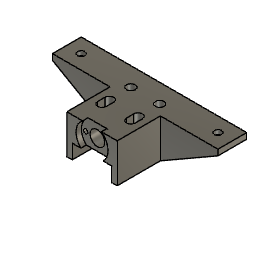
Z Carriage Bracket (Autodesk Fusion 360 design; units mm, degrees)
Autodesk Fusion 360 part; units mm, degrees
sketch "Sketch1" plane through (0, 0, 0) normal (0, 0, 1) x (1, 0, 0)
  line L0 (17.5, 25) -> (-17.5, 25)
  line L1 (-17.5, 25) -> (-17.5, -25)
  line L2 (-17.5, -25) -> (17.5, -25)
  line L3 (17.5, -25) -> (17.5, 25)
  line L4 (17.5, 25) -> (-17.5, -25) construction
  line L5 (-17.5, 25) -> (17.5, -25) construction
  line L6 (-13.7, 25) -> (13.7, 25)
  line L7 (13.7, 25) -> (13.7, -25)
  line L8 (13.7, -25) -> (-13.7, -25)
  line L9 (-13.7, -25) -> (-13.7, 25)
  line L10 (-57.5, 25) -> (57.5, 25)
  line L11 (57.5, 25) -> (57.5, 5)
  line L12 (57.5, 5) -> (-57.5, 5)
  line L13 (-57.5, 5) -> (-57.5, 25)
  line L14 (17.5, -8) -> (-17.5, -8) construction
  line L15 (17.5, 12) -> (-17.5, 12) construction
  line L16 (-10, -25) -> (-10, 25) construction
  line L17 (10, -25) -> (10, 26.6131) construction
  circle A0 centre (10, -8) radius 1.5
  circle A1 centre (10, 12) radius 1.5
  circle A2 centre (-10, 12) radius 1.5
  circle A3 centre (-10, -8) radius 1.5
  circle A4 centre (10, 12) radius 3
  circle A5 centre (-10, 12) radius 3
  circle A6 centre (-10, -8) radius 3
  circle A7 centre (10, -8) radius 3
  circle A8 centre (47.5, 15) radius 2.5
  circle A9 centre (47.5, 15) radius 4.5
  circle A10 centre (-47.5, 15) radius 2.5
  circle A11 centre (-47.5, 15) radius 4.5
  line L18 (-17.5, 21) -> (-57.5, 21)
  line L19 (-57.5, 21) -> (-57.5, 9)
  line L20 (-57.5, 9) -> (-17.5, 9)
  line L21 (-17.5, 9) -> (-17.5, 21)
  line L22 (57.5, 9) -> (17.5, 9)
  line L23 (17.5, 9) -> (17.5, 21)
  line L24 (17.5, 21) -> (57.5, 21)
  line L25 (57.5, 21) -> (57.5, 9)
  circle A12 centre (10, -3) radius 1.5
  circle A13 centre (10, -3) radius 3
  circle A14 centre (-10, -3) radius 3
  circle A15 centre (-10, -3) radius 1.5
  line L26 (-13, -8) -> (-13, -3)
  line L27 (-7, -8) -> (-7, -3)
  line L28 (7, -8) -> (7, -3)
  line L29 (13, -8) -> (13, -3)
  point P0 (-47.5, 15)
  point P1 (47.5, 15)
  dimension "d1" = 35
  dimension "d2" = 50
  dimension "d5" = 27.4
  dimension "d6" = 50
  dimension "d7" = 3.8
  dimension "d10" = 115
  dimension "d11" = 20
  dimension "d12" = 40
  dimension "d16" = 7.5
  dimension "d17" = 7.5
  dimension "d19" = 13
  dimension "d20" = 3
  dimension "d21" = 3
  dimension "d22" = 3
  dimension "d23" = 3
  dimension "d30" = 6
  dimension "d31" = 6
  dimension "d32" = 6
  dimension "d33" = 6
  dimension "d40" = 5
  dimension "d41" = 9
  dimension "d42" = 5
  dimension "d43" = 9
  dimension "d52" = 40
  dimension "d53" = 12
  dimension "d54" = 12
  dimension "d71" = 20
  dimension "d81" = 10
  dimension "d82" = 10
  dimension "d83" = 10
  dimension "d84" = 10
  dimension "d94" = 3
  dimension "d95" = 3
  dimension "d96" = 6
  dimension "d97" = 6
  dimension "d98" = 5
  constraint perpendicular L0 L1
  constraint parallel L0 L2
  constraint parallel L1 L3
  constraint horizontal L0
  constraint coincident L4 origin
  constraint coincident L5 origin
  constraint horizontal L6
  constraint vertical L7
  constraint horizontal L8
  constraint vertical L9
  constraint coincident L0 L6.start
  constraint horizontal L10
  constraint vertical L11
  constraint horizontal L12
  constraint vertical L13
  constraint coincident L0 L10.start
  constraint coincident L3 L14.start
  constraint coincident L1 L14.end
  constraint perpendicular L1 L14
  constraint coincident L3 L15.start
  constraint coincident L1 L15.end
  constraint perpendicular L1 L15
  constraint coincident L2 L16.start
  constraint coincident L0 L16.end
  constraint coincident L8 L17.start
  constraint perpendicular L10 L17
  constraint coincident L14 A0.centre
  constraint coincident L17 A0.centre
  constraint coincident L17 A1.centre
  constraint coincident L15 A1.centre
  constraint coincident L15 A2.centre
  constraint coincident L16 A2.centre
  constraint coincident L14 A3.centre
  constraint coincident L16 A3.centre
  constraint concentric A1 A4
  constraint concentric A2 A5
  constraint concentric A3 A6
  constraint concentric A0 A7
  constraint concentric A8 A9
  constraint concentric A10 A11
  constraint perpendicular L18 L19
  constraint parallel L18 L20
  constraint parallel L19 L21
  constraint horizontal L18
  constraint coincident P0 A10.centre
  constraint perpendicular L22 L23
  constraint parallel L22 L24
  constraint parallel L23 L25
  constraint horizontal L22
  constraint coincident P1 A8.centre
  constraint coincident L11 L22.start
  constraint concentric A14 A15
  constraint concentric A12 A13
  constraint coincident A6 L26.start
  constraint coincident L14 L26.start
  constraint coincident A14 L26.end
  constraint tangent A14 L26
  constraint perpendicular L14 L26
  constraint coincident A6 L27.start
  constraint coincident L14 L27.start
  constraint coincident A14 L27.end
  constraint tangent A14 L27
  constraint perpendicular L14 L27
  constraint coincident A7 L28.start
  constraint coincident L14 L28.start
  constraint coincident A13 L28.end
  constraint tangent A13 L28
  constraint perpendicular L14 L28
  constraint coincident A7 L29.start
  constraint coincident L14 L29.start
  constraint coincident A13 L29.end
  constraint tangent A13 L29
  constraint perpendicular L14 L29
  constraint horizontal A14.centre A12.centre
  measures "d1" distance of L1.end L2.end
  measures "d2" distance of L0.end L1.end
  measures "d5" distance of L6.start L6.end
  measures "d6" distance of L6.start L8.end
  measures "d7" distance of L1 L9
  measures "d10" distance of L10.start L10.end
  measures "d11" distance of L10.start L12.end
  measures "d12" distance of L3 L11
  measures "d16" distance of L3 L17
  measures "d17" distance of L1 L16
  measures "d19" distance of L10 L15
  measures "d20" diameter of A0
  measures "d21" diameter of A1
  measures "d22" diameter of A2
  measures "d23" diameter of A3
  measures "d30" diameter of A4
  measures "d31" diameter of A5
  measures "d32" diameter of A6
  measures "d33" diameter of A7
  measures "d40" diameter of A8
  measures "d41" diameter of A9
  measures "d42" diameter of A10
  measures "d43" diameter of A11
  measures "d52" distance of L19.end L20.end
  measures "d53" distance of L18.end L19.end
  measures "d54" distance of L22.end L23.end
  measures "d71" distance of L14 L15
  measures "d81" distance of L13 P0
  measures "d82" distance of L11 P1
  measures "d83" distance of L10 P1
  measures "d84" distance of L10 P0
  measures "d94" diameter of A12
  measures "d95" diameter of A15
  measures "d96" diameter of A14
  measures "d97" diameter of A13
  measures "d98" distance of A0.centre A12.centre
extrude "Extrude1" add sketch "Sketch1" along normal blind 27 contours L0 L3 L7 L10 L12 L23 | L0 L6 L7 L9 L10 L12 | L0 L1 L9 L10 L12 L21 | L2 L3 L7 L12 | L2 L7 L8 L9 L12 | L1 L2 L9 L12 | A0 | A1 | A2 | A3 | A4 | A5 | A6 A14 | A6 A14 L26 | A6 A14 L27 | A6 A14 | A6 A14 | A7 A13 | A7 A13 L28 | A7 A13 L29 | A7 A13 | A7 A13 | A12 | A15
extrude "Extrude2" cut sketch "Sketch1" along normal blind 10 contours L0 L6 L7 L9 L10 L12 | L2 L7 L8 L9 L12 | A0 | A1 | A2 | A3 | A4 | A5 | A6 A14 | A6 A14 L26 | A6 A14 L27 | A6 A14 | A6 A14 | A7 A13 | A7 A13 L28 | A7 A13 L29 | A7 A13 | A7 A13 | A12 | A15
extrude "Extrude3" add sketch "Sketch1" along normal blind 4 from surface at 23 contours L0 L3 L7 L10 L12 L23 | L3 L10 L11 L24 | L0 L6 L7 L9 L10 L12 | L3 L11 L22 L23 L24 L25 | L0 L1 L9 L10 L12 L21 | L3 L11 L12 L22 | L1 L10 L13 L18 | L1 L13 L18 L19 L20 L21 | L1 L12 L13 L20 | A1 | A2 | A4 | A5 | A8 | A9 | A10 | A11
extrude "Extrude6" cut sketch "Sketch1" along normal up to surface (13 mm away) from surface at 14 contours A0 | A3 | A6 A14 | A6 A14 L26 | A6 A14 L27 | A6 A14 | A6 A14 | A7 A13 | A7 A13 L28 | A7 A13 L29 | A7 A13 | A7 A13 | A12 | A15
extrude "Extrude7" cut sketch "Sketch1" along normal up to surface (13 mm away) from surface at 14 contours A1 | A2 | A4 | A5
extrude "Extrude4" cut sketch "Sketch1" along normal blind 3.8 from surface at 10 contours A0 | A3 | A12 | A15
extrude "Extrude5" cut sketch "Sketch1" along normal blind 3.8 from surface at 10 contours A1 | A2
extrude "Extrude8" cut sketch "Sketch1" along normal up to surface (4 mm away) from surface at 23 contours A8 | A10
extrude "Extrude9" cut sketch "Sketch1" along normal blind 1 from surface at 23 contours A8 | A9 | A10 | A11
extrude "Extrude10" add sketch "Sketch1" along normal up to surface (23 mm away) contours L3 L10 L11 L24 | L3 L11 L22 L23 L24 L25 | L3 L11 L12 L22 | L1 L10 L13 L18 | L1 L13 L18 L19 L20 L21 | L1 L12 L13 L20
sketch "Sketch2" plane through (0, -25, 0) normal (0, -1, 0) x (1, 0, 0)
  line L0 (-17.5, 0) -> (-17.5, 23)
  line L1 (17.5, 23) -> (17.5, 0)
  line L2 (-13.7, 0) -> (-13.7, 10)
  line L3 (-13.7, 10) -> (13.7, 10)
  line L4 (13.7, 10) -> (13.7, 0)
  line L5 (13.7, 0) -> (17.5, 0)
  line L6 (17.5, 0) -> (17.5, 27)
  line L7 (17.5, 27) -> (-17.5, 27)
  line L8 (-17.5, 27) -> (-17.5, 0)
  line L9 (-17.5, 0) -> (-13.7, 0)
  line L10 (17.5, 18) -> (-17.5, 18) construction
  line L11 (0, 23) -> (0, 10) construction
  circle A0 centre (0, 18) radius 5.125
  circle A1 centre (0, 18) radius 11.125
  line L12 (11.125, 18) -> (5.125, 18)
  line L13 (11.125, 18) -> (5.125, 18) construction
  line L14 (-5.125, 18) -> (-11.125, 18) construction
  circle A2 centre (-8.125, 18) radius 1.5
  circle A3 centre (8.125, 18) radius 1.5
  line L15 (-17.5, 27) -> (-57.5, 27)
  line L16 (-57.5, 27) -> (-57.5, 0)
  line L17 (-57.5, 0) -> (-17.5, 0)
  line L18 (-17.5, 0) -> (-17.5, 27)
  line L19 (17.5, 27) -> (57.5, 27)
  line L20 (57.5, 27) -> (57.5, 0)
  line L21 (57.5, 0) -> (17.5, 0)
  line L22 (17.5, 0) -> (17.5, 27)
  line L23 (-57.5, 27) -> (-17.5, 0) construction
  line L24 (-17.5, 27) -> (-57.5, 0) construction
  line L25 (17.5, 0) -> (57.5, 27) construction
  line L26 (17.5, 27) -> (57.5, 0) construction
  line L27 (-17.5, 23) -> (-57.5, 23)
  line L28 (-57.5, 23) -> (-57.5, 4)
  line L29 (-57.5, 4) -> (-17.5, 4)
  line L30 (-17.5, 4) -> (-17.5, 23)
  line L31 (-17.5, 23) -> (-57.5, 4) construction
  line L32 (-57.5, 23) -> (-17.5, 4) construction
  line L33 (57.5, 23) -> (17.5, 23)
  line L34 (17.5, 23) -> (17.5, 4)
  line L35 (17.5, 4) -> (57.5, 4)
  line L36 (57.5, 4) -> (57.5, 23)
  line L37 (57.5, 23) -> (17.5, 4) construction
  line L38 (17.5, 23) -> (57.5, 4) construction
  line L39 (-17.5, 0) -> (-57.5, 23)
  line L40 (17.5, 0) -> (57.5, 23)
  point P0 (-37.5, 13.5)
  point P1 (37.5, 13.5)
  dimension "d64" = 8
  dimension "d65" = 10.25
  dimension "d66" = 22.25
  dimension "d74" = 3
  dimension "d75" = 3
  dimension "d85" = 40
  dimension "d86" = 27
  dimension "d87" = 40
  dimension "d88" = 27
  dimension "d89" = 19
  dimension "d90" = 40
  dimension "d91" = 19
  constraint coincident L1 L10.start
  constraint coincident L8 L10.end
  constraint perpendicular L8 L10
  constraint midpoint L3 L11.end
  constraint midpoint L10 A0.centre
  constraint concentric A0 A1
  constraint coincident L10 L12.start
  constraint coincident A1 L12.start
  constraint coincident L10 L12.end
  constraint coincident A0 L12.end
  constraint parallel L12 L13
  constraint coincident L10 L14.start
  constraint coincident A0 L14.start
  constraint coincident A1 L14.end
  constraint coincident L10 L14.end
  constraint midpoint L14 A2.centre
  constraint midpoint L12 A3.centre
  constraint horizontal L15
  constraint vertical L16
  constraint horizontal L17
  constraint vertical L18
  constraint coincident L7.end L8.start
  constraint horizontal L19
  constraint vertical L20
  constraint horizontal L21
  constraint vertical L22
  constraint coincident L6.end L7.start
  constraint perpendicular L27 L28
  constraint parallel L27 L29
  constraint parallel L28 L30
  constraint horizontal L27
  constraint coincident L31 P0
  constraint coincident L32 P0
  constraint midpoint L23 P0
  constraint perpendicular L33 L34
  constraint parallel L33 L35
  constraint parallel L34 L36
  constraint horizontal L33
  constraint coincident L37 P1
  constraint coincident L38 P1
  constraint midpoint L25 P1
  constraint coincident L0.start L8.end
  measures "d64" distance of L3 L10
  measures "d65" diameter of A0
  measures "d66" diameter of A1
  measures "d74" diameter of A2
  measures "d75" diameter of A3
  measures "d85" distance of L7.end L15.end
  measures "d86" distance of L7.end L0.start
  measures "d87" distance of L6.end L19.end
  measures "d88" distance of L6.end L1.end
  measures "d89" distance of L27.end L28.end
  measures "d90" distance of L34.end L35.end
  measures "d91" distance of L1.start L34.end
extrude "Extrude16" cut sketch "Sketch2" against normal up to surface (50 mm away) contours L16 L17 L29 L39 | L16 L28 L29 L39 | L20 L21 L35 L40 | L20 L35 L36 L40
extrude "Extrude14" cut sketch "Sketch2" against normal blind 3.75 contours L3 L7 A1 | A0 | L12 A3 | L12 A3 | A2
extrude "Extrude13" cut sketch "Sketch2" against normal up to surface (50 mm away) contours A0
extrude "Extrude15" cut sketch "Sketch2" against normal blind 5 from surface at -3.75 contours L12 A3 | L12 A3 | A2
extrude "Extrude11" cut sketch "Sketch1" along normal up to surface (19 mm away) from surface at 4 contours L3 L11 L22 L23 L24 L25 | L1 L13 L18 L19 L20 L21
